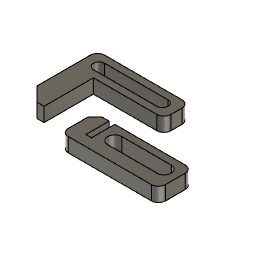
server-top-holders (Autodesk Fusion 360 design; units mm, degrees)
Autodesk Fusion 360 part; units mm, degrees
sketch "back" plane through (0, 0, 0) normal (0, 0, 1) x (1, 0, 0)
  line L0 (-37.1625, 9.7554) -> (-37.1625, 62.9)
  line L1 (-37.1625, 62.9) -> (27.8375, 62.9)
  line L2 (27.8375, 62.9) -> (27.8375, 45)
  line L3 (27.8375, 45) -> (-22.1625, 45)
  line L4 (-22.1625, 45) -> (-22.1625, 10)
  line L5 (-22.1625, 10) -> (-37.1625, 10)
  line L6 (-37.1625, 10) -> (-37.1625, 9.7554)
  line L7 (27.8375, 53.95) -> (-37.1625, 53.95) construction
  line L8 (17.8375, 62.9) -> (17.8375, 53.95)
  line L9 (-27.1625, 62.9) -> (-27.1625, 53.95)
  line L10 (-27.1625, 50) -> (17.8375, 50)
  arc A0 (17.8375, 50) -> (17.8375, 57.9) centre (17.8375, 53.95) ccw
  line L11 (17.8375, 57.9) -> (-27.1625, 57.9)
  arc A1 (-27.1625, 57.9) -> (-27.1625, 50) centre (-27.1625, 53.95) ccw
  line L12 (-27.1625, 53.95) -> (17.8375, 53.95) construction
  line L13 (0, 0) -> (-32, 0) construction
  line L14 (0, 0) -> (0, 18) construction
  line L15 (-22.1625, 45) -> (-37.1625, 45)
  point P0 (-27.1625, 53.95)
  point P1 (17.8375, 53.95)
  dimension "d1" = 10
  dimension "d2" = 10
  dimension "d3" = 35
  dimension "d5" = 15
  dimension "d6" = 7.9
  dimension "d7" = 45
  dimension "d8" = 5
  dimension "d9" = 10
  dimension "d10" = 22.1625
  constraint vertical L0
  constraint perpendicular L0 L1
  constraint perpendicular L1 L2
  constraint perpendicular L2 L3
  constraint perpendicular L3 L4
  constraint perpendicular L2 L5
  constraint perpendicular L5 L6
  constraint midpoint L2 L7.start
  constraint coincident L0 L7.end
  constraint perpendicular L0 L7
  constraint coincident L1 L8.start
  constraint coincident L7 P1
  constraint perpendicular L7 L8
  constraint coincident L1 L9.start
  constraint coincident L7 P0
  constraint perpendicular L7 L9
  constraint coincident P0 L9.end
  constraint coincident P1 L8.end
  constraint tangent L10 A0
  constraint tangent A0 L11
  constraint parallel L10 L11
  constraint tangent L11 A1
  constraint tangent L10 A1
  constraint perpendicular L8 L12
  constraint coincident L13.start L14.start
  constraint horizontal L13
  constraint perpendicular L13 L14
  constraint coincident L0 L15.end
  constraint perpendicular L0 L15
  measures "d1" distance of L0 L9
  measures "d2" distance of L2 L8
  measures "d3" distance of L3.end L4.end
  measures "d5" distance of L4.end L5.end
  measures "d6" diameter of A0
  measures "d7" distance of A0.end L11.end
  measures "d8" distance of L3 L10
  measures "d9" distance of L5 L13
  measures "d10" distance of L4 L14
  measures "d35" distance of L3.end
extrude "Extrude1" add sketch "back" along normal blind 10 contours L0 L4 L5 L15 | L0 L1 L2 L3 L8 L9 L10 A0 A1 L15 | L1 L8 L9 L11 makes body 1
chamfer "Chamfer1" distance 10 angle 45 1 edges at (-37.1625, 10, 5) on bodies 1
fillet "Fillet1" radius 5 tangency weight 0.95723 3 edges at (-37.1625, 62.9, 5) (27.8375, 62.9, 5) (27.8375, 45, 5) on bodies 1
sketch "front" plane through (0, 0, 0) normal (0, 0, 1) x (1, 0, 0)
  line L0 (0, 24) -> (10, 24)
  line L1 (10, 24) -> (10, 7.5)
  line L2 (10, 7.5) -> (14, 7.5)
  line L3 (14, 7.5) -> (14, 24)
  line L4 (0, 0) -> (69, 0)
  line L5 (0, 24) -> (0, 0)
  line L6 (14, 14) -> (69, 14) construction
  line L7 (24, 9) -> (59, 9)
  arc A0 (59, 9) -> (59, 19) centre (59, 14) ccw
  line L8 (59, 19) -> (24, 19)
  arc A1 (24, 19) -> (24, 9) centre (24, 14) ccw
  line L9 (24, 14) -> (59, 14) construction
  line L10 (14, 24) -> (69, 24)
  line L11 (69, 24) -> (69, 0)
  point P0 (19, 14)
  point P1 (64, 14)
  dimension "d27" = 10
  dimension "d28" = 16.5
  dimension "d35" = 4
  dimension "d55" = 7.5
  dimension "d56" = 10
  dimension "d58" = 5
  dimension "d59" = 5
  dimension "d60" = 35
  dimension "d65" = 5
  constraint perpendicular L0 L1
  constraint perpendicular L1 L2
  constraint perpendicular L2 L3
  constraint equal L1 L3
  constraint vertical L5
  constraint parallel L0 L6
  constraint tangent L7 A0
  constraint tangent A0 L8
  constraint parallel L7 L8
  constraint tangent L8 A1
  constraint tangent L7 A1
  constraint coincident L6 A0.centre
  constraint parallel L6 L9
  constraint horizontal L10
  constraint midpoint A1 P0
  constraint midpoint A0 P1
  constraint horizontal P0 P1
  constraint coincident L6.end L11
  constraint coincident L4.start L5.end
  constraint perpendicular L10 L11
  constraint coincident L3 L6.start
  measures "d27" distance of L0.start L0.end
  measures "d28" distance of L0.end L1.end
  measures "d35" distance of L1.end L2.end
  measures "d55" distance of L2 L4
  measures "d56" diameter of A0
  measures "d58" distance of L6.start P0
  measures "d59" distance of L6.end P1
  measures "d60" distance of A0.end L8.end
  measures "d65" distance of L8 L10
extrude "Extrude4" add sketch "front" along normal blind 10 separate body makes body 2
fillet "Fillet4" radius 5 3 edges at (69, 0, 5) (0, 0, 5) (69, 24, 5) on bodies 2
chamfer "Chamfer4" distance 5 angle 45 1 edges at (0, 24, 5) on bodies 2
named bodies: "server-holder-back", "server-holder-front"
